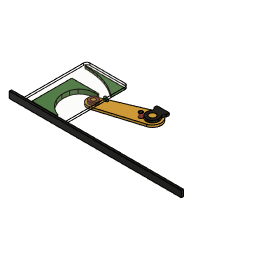
Arpione - Metodo Geometrico [NEW] v2 (Autodesk Fusion 360 design; units mm, degrees)
Autodesk Fusion 360 part; units mm, degrees
sketch "Manovella + Catena" plane through (0, 0, 0) normal (0, 0, 1) x (1, 0, 0)
  circle A0 centre (0, 0) radius 14.5
  line L0 (0, 0) -> (-101.6567, -37)
  circle A1 centre (-101.6567, -37) radius 10
  circle A2 centre (-101.6567, -37) radius 15
  circle A3 centre (0, 0) radius 20.5
  line L1 (-107.497, -23.1837) -> (-7.9817, 18.8823)
  line L2 (-97.2496, -51.338) -> (6.023, -19.5953)
  circle A4 centre (-101.6567, -37) radius 5
  circle A5 centre (0, 0) radius 7.5
  line L3 (-38.7092, -123.6808) -> (196.3889, -123.6808)
  line L4 (-38.7092, -128.6808) -> (196.3889, -128.6808)
  line L5 (196.3889, -128.6808) -> (196.3889, -123.6808)
  line L6 (-99.9998, -123.6808) -> (-207.841, -123.6808)
  line L7 (-207.841, -128.6808) -> (-207.841, -123.6808)
  line L8 (0, 0) -> (6.023, -19.5953) construction
  line L9 (-7.9817, 18.8823) -> (0, 0) construction
  line L10 (0, 0) -> (0, 20.5) construction
  line L11 (-99.9998, -123.6808) -> (-99.9998, -128.6808) construction
  line L12 (-207.841, -128.6808) -> (-99.9998, -128.6808)
  line L13 (-99.9998, -123.6808) -> (-38.7092, -123.6808)
  line L14 (-38.7092, -123.6808) -> (-38.7092, -128.6808) construction
  line L15 (-99.9998, -128.6808) -> (-38.7092, -128.6808)
  line L16 (0, 0) -> (-0.6635, -0.2415)
  line L17 (0, 0) -> (-15.5734, -11.7354)
  circle A6 centre (-15.5734, -11.7354) radius 2.5
  circle A7 centre (-15.5734, -11.7354) radius 4.5
  line L18 (-52.6515, 0) -> (0, 0) construction
  circle A8 centre (-101.6567, -37) radius 13 construction
  line L19 (0, 0) -> (0, -19.5) construction
  circle A9 centre (0, -19.5) radius 4.5 construction
  line L20 (0, -24) -> (-101.6567, -24) construction
  line L21 (-101.6567, -37) -> (-115.7521, -42.1303) construction
  circle A10 centre (0, 0) radius 123.1808 construction
  line L22 (0.0515, -123.1808) -> (0.0515, -123.6808)
  dimension "d1" = 29
  dimension "d8" = 20
  dimension "d43" = 0
  dimension "d44" = 0
  dimension "d45" = 0
  dimension "d46" = 0
  dimension "d197" = 5
  dimension "d198" = 6
  dimension "d199" = -5
  dimension "d200" = -7
  dimension "d312" = 5
  dimension "d449" = 23.372
  dimension "d648" = 19.5
  dimension "d650" = 17
  dimension "d651" = 5
  dimension "d653" = 9
  dimension "d654" = 20
  dimension "d655" = 3
  dimension "d656" = 85.4786
  dimension "d658" = 0.5
  constraint coincident A0.centre L0.start
  constraint coincident L0.end A1.centre
  constraint coincident A2 L1.start
  constraint coincident A3 L1.end
  constraint tangent A3 L1
  constraint tangent A2 L1
  constraint coincident A2 L2.start
  constraint coincident A3 L2.end
  constraint tangent A3 L2
  constraint tangent A2 L2
  constraint perpendicular L3 L5
  constraint coincident L3 L13.end
  constraint horizontal L3
  constraint horizontal L4
  constraint perpendicular L6 L7
  constraint coincident A3 L10.end
  constraint vertical L10
  constraint perpendicular L4 L11
  constraint horizontal L12
  constraint perpendicular L4 L14
  constraint horizontal L15
  constraint coincident L0 L16.end
  constraint coincident L17.end A6.centre
  constraint concentric A6 A7
  constraint horizontal L18
  constraint coincident L1 L18.start
  constraint vertical L19
  constraint equal L17 L19
  constraint coincident L19.end A9.centre
  constraint equal A7 A9
  constraint horizontal L20
  constraint tangent A9 L20
  constraint coincident A9 L20.start
  constraint tangent A8 L20
  constraint coincident A8 L20.end
  constraint coincident A2 L21.end
  constraint collinear L0 L21
  constraint coincident L21.end A10
  constraint coincident A10 L22.start
  constraint coincident L3 L22.end
  constraint perpendicular L3 L22
  measures "d1" diameter of A0
  measures "d8" diameter of A1
  measures "d312" distance of L3.end L4.end
  measures "d540" distance of A0.centre
  measures "d648" distance of A0.centre L17.end
  measures "d650" angle of L0 L17
  measures "d651" diameter of A6
  measures "d653" diameter of A7
  measures "d654" angle of L0 L18
  measures "d658" distance of L22.start L22.end
sketch "Curva Principale" plane through (0, 0, 0) normal (0, 0, 1) x (1, 0, 0)
  circle A0 centre (0, 0) radius 14.5
  circle A1 centre (-101.6567, -37) radius 10
  line L0 (0, 0) -> (-101.6567, -37)
  line L1 (0, 0) -> (-300, 0) construction
  line L2 (-10, 0) -> (-111.5208, -37.3713) construction
  line L3 (-20, 0) -> (-120.62, -39.7327) construction
  line L4 (-30, 0) -> (-128.2041, -45.3766) construction
  line L5 (-40, 0) -> (-133.2404, -54.8571) construction
  line L6 (-50, 0) -> (-134.4276, -67.6392) construction
  line L7 (-60, 0) -> (-130.2578, -82.2613) construction
  line L8 (-70, 0) -> (-119.9523, -95.9575) construction
  line L9 (-80, 0) -> (-103.6726, -105.5589) construction
  circle A2 centre (-111.5208, -37.3713) radius 10 construction
  circle A3 centre (-120.62, -39.7327) radius 10 construction
  circle A4 centre (-128.2041, -45.3766) radius 10 construction
  circle A5 centre (-133.2404, -54.8571) radius 10 construction
  circle A6 centre (-134.4276, -67.6392) radius 10 construction
  circle A7 centre (-130.2578, -82.2613) radius 10 construction
  circle A8 centre (-119.9523, -95.9575) radius 10 construction
  circle A9 centre (-103.6726, -105.5589) radius 10 construction
  line L10 (-165.6808, -117.9148) -> (-165.6808, 0)
  line L11 (-101.6567, -37) -> (-92.2597, -33.5798) construction
  line L12 (-101.6567, -37) -> (-105.0769, -27.6031) construction
  line L13 (-111.5208, -37.3713) -> (-114.9753, -27.9869) construction
  line L14 (-111.5208, -37.3713) -> (-120.9051, -40.8258) construction
  line L15 (-120.62, -39.7327) -> (-129.9211, -43.4055) construction
  line L16 (-120.62, -39.7327) -> (-124.2928, -30.4316) construction
  line L17 (-128.2041, -45.3766) -> (-137.2818, -49.5712) construction
  line L18 (-133.2404, -54.8571) -> (-141.8594, -59.9279) construction
  line L19 (-133.2404, -54.8571) -> (-138.3113, -46.2381) construction
  line L20 (-134.4276, -67.6392) -> (-142.2319, -73.8917) construction
  line L21 (-134.4276, -67.6392) -> (-140.68, -59.8349) construction
  line L22 (-130.2578, -82.2613) -> (-136.7523, -89.8654) construction
  line L23 (-130.2578, -82.2613) -> (-137.8618, -75.7668) construction
  line L24 (-119.9523, -95.9575) -> (-109.1547, -75.2156) construction
  line L25 (-109.1547, -75.2156) -> (-124.5698, -104.8276) construction
  line L26 (-119.9523, -95.9575) -> (-128.8224, -91.34) construction
  line L27 (-103.6726, -105.5589) -> (-105.8608, -115.3166) construction
  line L28 (-103.6726, -105.5589) -> (-113.4302, -103.3707) construction
  line L29 (-128.2041, -45.3766) -> (-132.3986, -36.2989) construction
  line L30 (-102.4867, -27.0345) -> (-102.4867, -23.9148)
  line L31 (-102.4867, -23.9148) -> (-165.6808, -23.9148)
  line L32 (-107.506, -117.9148) -> (-165.6808, -117.9148)
  spline S0 degree 5 poles (-102.4867, -27.0345) (-102.9803, -27.0181) (-103.9715, -26.994) (-105.4699, -26.9842) (-107.4912, -27.0236) (-110.0566, -27.1642) (-112.6596, -27.4066) (-115.2977, -27.7716) (-117.9665, -28.2935) (-120.6573, -29.0126) (-123.3546, -29.9669) (-126.0334, -31.1852) (-128.6561, -32.6772) (-131.1759, -34.4349) (-133.5437, -36.4389) (-135.715, -38.6632) (-137.6558, -41.081) (-139.3501, -43.6698) (-140.7956, -46.4106) (-141.9983, -49.2867) (-142.9681, -52.2823) (-143.7134, -55.3813) (-144.2371, -58.5657) (-144.538, -61.8174) (-144.6118, -65.1181) (-144.4531, -68.4506) (-144.0563, -71.7998) (-143.4169, -75.1531) (-142.532, -78.4992) (-141.4009, -81.8266) (-140.0249, -85.1225) (-138.4082, -88.3709) (-136.5584, -91.5515) (-134.4857, -94.6403) (-132.202, -97.6115) (-129.7196, -100.4395) (-127.0505, -103.101) (-124.2053, -105.5765) (-121.1919, -107.8525) (-118.0161, -109.9209) (-114.6816, -111.7773) (-111.889, -113.0913) (-109.7246, -113.9805) (-108.2507, -114.5306) (-107.506, -114.795) knots 0 0 0 0 0 0 0.025 0.05 0.075 0.1 0.125 0.15 0.175 0.2 0.225 0.25 0.275 0.3 0.325 0.35 0.375 0.4 0.425 0.45 0.475 0.5 0.525 0.55 0.575 0.6 0.625 0.65 0.675 0.7 0.725 0.75 0.775 0.8 0.825 0.85 0.875 0.9 0.925 0.95 0.975 1 1 1 1 1 1
  line L33 (-102.4867, -27.0345) -> (-165.6808, -27.0345) construction
  line L34 (-107.506, -114.795) -> (-107.506, -117.9148)
  line L35 (-107.506, -114.795) -> (-165.6808, -114.795) construction
  line L36 (-102.4867, -27.0345) -> (-101.6567, -37) construction
  line L37 (-112.7142, -27.4428) -> (-111.5208, -37.3713) construction
  line L38 (-135.8335, -38.9121) -> (-128.2041, -45.3766)
  line L39 (-142.8322, -52.029) -> (-133.2404, -54.8571)
  line L40 (-144.4026, -68.3455) -> (-134.4276, -67.6392)
  line L41 (-130.2578, -82.2613) -> (-139.4301, -86.2449)
  line L42 (-119.9523, -95.9575) -> (-126.7298, -103.3105)
  line L43 (-107.506, -114.795) -> (-103.6726, -105.5589)
  point P0 (-10, 0)
  point P1 (-20, 0)
  point P2 (-30, 0)
  point P3 (-40, 0)
  point P4 (-50, 0)
  point P5 (-60, 0)
  point P6 (-70, 0)
  point P7 (-80, 0)
  point P8 (-112.7142, -27.4428)
  point P9 (-124.2928, -30.4316)
  point P10 (-135.8335, -38.9121)
  point P11 (-142.8322, -52.029)
  point P12 (-144.4026, -68.3455)
  point P13 (-139.4301, -86.2449)
  point P14 (-126.7298, -103.3105)
  dimension "d616" = 10
  dimension "d617" = 10
  dimension "d618" = 10
  dimension "d619" = 10
  dimension "d620" = 10
  dimension "d621" = 10
  dimension "d622" = 10
  dimension "d623" = 10
  dimension "d625" = 20
  dimension "d626" = 20.209
  dimension "d627" = 21.548
  dimension "d628" = 24.8
  dimension "d629" = 30.47
  dimension "d630" = 38.7
  dimension "d631" = 49.5
  dimension "d632" = 62.5
  dimension "d633" = 77.36
  dimension "d686" = 94
  constraint coincident A0.centre L0.start
  constraint horizontal L1
  constraint coincident L1 P0
  constraint coincident L1 P1
  constraint coincident L1 P2
  constraint coincident L1 P3
  constraint coincident L1 P4
  constraint coincident L1 P5
  constraint coincident L1 P6
  constraint coincident L1 P7
  constraint coincident P0 L2.start
  constraint coincident P1 L3.start
  constraint coincident P2 L4.start
  constraint coincident P3 L5.start
  constraint coincident P4 L6.start
  constraint coincident P5 L7.start
  constraint coincident P6 L8.start
  constraint coincident P7 L9.start
  constraint equal L0 L2
  constraint equal L2 L3
  constraint equal L3 L4
  constraint equal L4 L5
  constraint equal L5 L6
  constraint equal L6 L7
  constraint equal L7 L8
  constraint equal L8 L9
  constraint coincident L2.end A2.centre
  constraint coincident L3.end A3.centre
  constraint coincident L4.end A4.centre
  constraint coincident L5.end A5.centre
  constraint coincident L6.end A6.centre
  constraint coincident L7.end A7.centre
  constraint coincident L8.end A8.centre
  constraint coincident L9.end A9.centre
  constraint equal A1 A2
  constraint equal A2 A3
  constraint equal A3 A4
  constraint equal A4 A5
  constraint equal A5 A6
  constraint equal A6 A7
  constraint equal A7 A8
  constraint equal A8 A9
  constraint coincident L1 L10.end
  constraint vertical L10
  constraint coincident A1.centre L0.end
  constraint coincident A1 L11.end
  constraint coincident A2 L13.end
  constraint coincident A2 L14.end
  constraint coincident A3 L15.end
  constraint coincident A3 P9
  constraint coincident A4 L17.end
  constraint coincident A5 L18.end
  constraint coincident A5 L19.end
  constraint coincident A6 L20.end
  constraint coincident A6 L21.end
  constraint coincident A7 L22.end
  constraint coincident A7 L23.end
  constraint coincident A8 L25.end
  constraint coincident A8 L26.end
  constraint coincident A9 L27.end
  constraint coincident A9 L28.end
  constraint collinear L0 L11
  constraint collinear L2 L14
  constraint collinear L3 L15
  constraint collinear L4 L17
  constraint collinear L5 L18
  constraint collinear L6 L20
  constraint collinear L7 L22
  constraint collinear L8 L25
  constraint collinear L9 L27
  constraint perpendicular L27 L28
  constraint perpendicular L25 L26
  constraint perpendicular L22 L23
  constraint perpendicular L20 L21
  constraint perpendicular L18 L19
  constraint perpendicular L15 L16
  constraint coincident A4 L29.end
  constraint perpendicular L17 L29
  constraint perpendicular L13 L14
  constraint perpendicular L11 L12
  constraint coincident L10 L31.end
  constraint perpendicular L10 L31
  constraint coincident L10.start L32.end
  constraint coincident A1 L12.end
  constraint coincident A2 P8
  constraint coincident A4 P10
  constraint coincident A5 P11
  constraint coincident A6 P12
  constraint coincident A7 P13
  constraint coincident A8 P14
  constraint coincident A9 S0.end
  constraint coincident A1 L30.start
  constraint coincident L10 L33.end
  constraint perpendicular L10 L33
  constraint perpendicular L32 L34
  constraint coincident L10 L35.end
  constraint perpendicular L10 L35
  constraint equal L30 L34
  constraint vertical L30
  constraint vertical L34
  constraint coincident P8 L37.start
  constraint coincident P10 L38.start
  constraint coincident P11 L39.start
  constraint coincident P12 L40.start
  constraint coincident P13 L41.end
  constraint coincident P14 L42.end
  measures "d616" distance of A0.centre P0
  measures "d617" distance of P0 P1
  measures "d618" distance of P1 P2
  measures "d619" distance of P2 P3
  measures "d620" distance of P3 P4
  measures "d621" distance of P4 P5
  measures "d622" distance of P5 P6
  measures "d623" distance of P6 P7
  measures "d625" angle of L0 L1
  measures "d626" angle of L1 L2
  measures "d627" angle of L1 L3
  measures "d628" angle of L1 L4
  measures "d629" angle of L1 L5
  measures "d630" angle of L1 L6
  measures "d631" angle of L1 L7
  measures "d632" angle of L1 L8
  measures "d633" angle of L1 L9
  measures "d686" distance of L10.start L31.end
sketch "Curva secondaria" plane through (0, 0, 0) normal (0, 0, 1) x (1, 0, 0)
  line L0 (-100.0056, -0.0109) -> (0, 0.0109)
  circle A0 centre (-88.1799, -15.52) radius 4.5 construction
  line L1 (-80, 0) -> (-78.5176, -19.4436) construction
  circle A1 centre (-78.5176, -19.4436) radius 4.5 construction
  line L2 (-88.1799, -15.52) -> (-100, -0.0109) construction
  line L3 (-80, 0) -> (-103.6726, -105.5589)
  circle A2 centre (-103.6726, -105.5589) radius 10
  line L4 (-90, -0.0087) -> (-83.167, -18.2723) construction
  circle A3 centre (-83.167, -18.2723) radius 4.5 construction
  line L5 (-91.4991, -20.02) -> (-88.1799, -20.02) construction
  line L6 (-91.4815, -23.9436) -> (-78.5176, -23.9436) construction
  circle A4 centre (-15.5734, -11.7354) radius 4.5
  line L7 (0, 0) -> (-15.5734, -11.7354)
  line L8 (-91.5063, -22.7723) -> (-83.167, -22.7723) construction
  line L9 (-83.167, -18.2723) -> (-81.5901, -22.487) construction
  line L10 (-83.167, -18.2723) -> (-87.3817, -19.8492) construction
  line L11 (-88.1799, -15.52) -> (-85.4521, -19.0991) construction
  line L12 (-88.1799, -15.52) -> (-91.7589, -18.2478) construction
  arc A5 (-89.8544, -20.02) -> (-79.0195, -23.9436) centre (-84.6752, -22.6399) ccw
  line L13 (-89.8544, -20.02) -> (-84.2048, -22.7723)
  line L14 (-84.2048, -22.7723) -> (-79.0195, -23.9436)
  line L15 (-78.5176, -19.4436) -> (-78.1754, -23.9305) construction
  line L16 (-78.5176, -19.4436) -> (-83.0045, -19.7857) construction
  point P0 (-100, -0.0109)
  point P1 (-90, -0.0087)
  dimension "d536" = 127.3
  dimension "d638" = 73.708
  dimension "d639" = 10
  dimension "d641" = 10
  dimension "d642" = 110.5
  dimension "d649" = 17
  dimension "d657" = 36.988
  constraint coincident L1.end A1.centre
  constraint coincident L1.start L3.start
  constraint coincident A0.centre L2.start
  constraint coincident P0 L2.end
  constraint coincident L0 P0
  constraint coincident L0 P1
  constraint coincident P1 L4.start
  constraint equal L1 L4
  constraint coincident L4.end A3.centre
  constraint equal A1 A3
  constraint equal A0 A3
  constraint equal L2 L4
  constraint horizontal L5
  constraint horizontal L6
  constraint tangent A1 L6
  constraint tangent A0 L5
  constraint horizontal L8
  constraint tangent A3 L8
  constraint coincident A3 L8.end
  constraint coincident A0 L5.end
  constraint coincident A1 L6.end
  constraint coincident A3 L9.end
  constraint parallel L4 L9
  constraint coincident A3 L10.end
  constraint perpendicular L9 L10
  constraint coincident A0 L11.end
  constraint collinear L2 L11
  constraint coincident A0 L12.end
  constraint perpendicular L11 L12
  constraint coincident L6 A5.end
  constraint equal A1 A4
  constraint equal L1 L7
  constraint coincident L5 A5.start
  constraint coincident L8 L13.end
  constraint tangent A3 L13
  constraint tangent A1 L14
  constraint coincident A1 L15.end
  constraint coincident A1 L16.end
  constraint perpendicular L1 L16
  measures "d536" angle of L0 L2
  measures "d639" horizontal distance of L1.start P1
  measures "d641" horizontal distance of P0 P1
  measures "d642" angle of L0 L4
  measures "d649" angle of L1 L3
  measures "d657" angle of L0 L7
extrude "Extrude1" add sketch "Curva Principale" along normal blind 10 contours L10 L30 L31 L32 S0 L34 makes body 1 in component "Arpione_Curva1"
fillet "Fillet12" radius 0.4 2 edges at (-102.4867, -27.0345, 5) (-107.506, -114.795, 5) on bodies 1 in component "Arpione_Curva1"
extrude "Extrude1'" add sketch "Manovella + Catena" against normal blind 5 separate body contours A0 L0 A5 L17 | A0 L0 A3 L17 A7 | A0 L0 A5 L17 | A0 L0 A3 L17 A7 | L0 A5 L16 L17 | L0 A5 L16 L17 | L0 A2 A3 L2 A7 | L0 A2 A3 L1 | A3 L17 A6 A7 | A3 L17 A6 A7 | A2 | A3 A6 A7 | A3 A6 | A3 A6 | A1 | A4 makes body 2 in component "Manopola"
extrude "Extrude2" add sketch "Manovella + Catena" along normal blind 5 contours A4 bodies 2 in component "Manopola"
extrude "Extrude3" add sketch "Manovella + Catena" against normal blind 10 contours L0 A5 L16 L17 | L0 A5 L16 L17 bodies 2 in component "Manopola"
extrude "Extrude4" add sketch "Manovella + Catena" along normal blind 10 contours A3 A6 | A3 A6 bodies 2 in component "Manopola"
extrude "Extrude5" add sketch "Manovella + Catena" along normal blind 5 contours L0 A5 L16 L17 | L0 A5 L16 L17 bodies 2 in component "Manopola"
sketch "Fulcro" plane through (0, 0, 0) normal (0, 0, 1) x (1, 0, 0)
  circle A0 centre (0, 0) radius 14.5
  circle A1 centre (0, 0) radius 7.5
  line L0 (0, 0) -> (-14.5, 0)
  line L1 (0, 0) -> (14.5, 0)
  line L2 (14.5, 0) -> (14.5, 25)
  line L3 (14.5, 25) -> (-14.5, 25)
  line L4 (-14.5, 25) -> (-14.5, 0)
  line L5 (-15.5734, -11.7354) -> (0, 0)
  line L6 (0, 0) -> (15.5734, 11.7354) construction
  circle A2 centre (15.5734, 11.7354) radius 4.5 construction
  arc A3 (14.5, 17.9188) -> (14.5, 6.5018) centre (17.4303, 12.2103) ccw
  line L7 (0, 0) -> (0, 14.5) construction
  circle A4 centre (-15.5734, -11.7354) radius 4.5
  arc A5 (14.5, 0) -> (12.1494, 8.5653) centre (-2.2808, 0) ccw
  arc A6 (-14.5, 6.5018) -> (-14.5, 17.9188) centre (-17.4303, 12.2103) ccw
  arc A7 (-12.1494, 8.5653) -> (-14.5, 0) centre (2.2808, 0) ccw
  dimension "d540" = 25
  constraint coincident A0.centre A1.centre
  constraint coincident A0 L0.end
  constraint horizontal L0
  constraint coincident A0 L1.end
  constraint horizontal L1
  constraint perpendicular L1 L2
  constraint perpendicular L2 L3
  constraint tangent A0 L4
  constraint coincident L5.start A4.centre
  constraint parallel L5 L6
  constraint equal L5 L6
  constraint coincident L6.end A2.centre
  constraint equal A2 A4
  constraint tangent A2 A3
  constraint coincident L2 A3.end
  constraint coincident L2 A3.start
  constraint coincident A0 L7.end
  constraint vertical L7
  constraint tangent L2 A5
  constraint coincident A3 A5.end
  constraint symmetric L1.end L7 L0.end
  constraint symmetric A3.start L7 A6.end
  constraint symmetric A3.end L7 A6.start
  constraint symmetric A3 L7 A6
  constraint symmetric L7 A5.end A7.start
  constraint symmetric L7 A5 A7
  measures "d540" distance of L1.end L2.end
extrude "Extrude1''" add sketch "Fulcro" along normal blind 5 separate body contours A0 A1 L0 L1 | A0 A1 L1 L5 | A0 L2 L3 L4 A3 A5 A6 A7 | A0 A1 L0 L5 makes body 3 in component "Fulcro"
extrude "Extrude1'''" add sketch "Manovella + Catena" along normal blind 5 separate body contours A1 makes body 4 in component "Cuscinetto_Basso"
extrude "Extrude1''''" add sketch "Manovella + Catena" along normal blind 10 separate body contours A3 L17 A6 A7 | A3 L17 A6 A7 | A3 A6 A7 makes body 5 in component "Cuscinetto_Alto"
extrude "Extrude1'''''" add sketch "Manovella + Catena" along normal blind 15 separate body contours L3 L4 L5 L6 L7 L12 L13 L15 makes body 6 in component "Catena"
extrude "Extrude1''''''" add sketch "Curva secondaria" along normal blind 4 from surface at 6 separate body contours L3 A5 L13 L14 | L3 A5 L13 makes body 7 in component "Arpione_Curva2"
sketch "Curva Frenante" plane through (0, 0, 0) normal (0, 0, 1) x (1, 0, 0)
  circle A0 centre (0, 0) radius 14.5
  line L0 (-88.1799, -15.52) -> (-100, -0.0109) construction
  circle A1 centre (-88.1799, -15.52) radius 4.5
  line L1 (0, 0) -> (-300, 0) construction
  line L2 (-110, 0) -> (-94.2042, -11.4343) construction
  line L3 (-120, 0) -> (-101.6528, -6.6054) construction
  line L4 (-130, 0) -> (-110.5713, -1.6656) construction
  line L5 (-140, 0) -> (-120.6898, 2.7139) construction
  line L6 (-150, 0) -> (-131.5294, 6.252) construction
  line L7 (-160, 0) -> (-142.6099, 8.8225) construction
  line L8 (-170, 0) -> (-153.5539, 10.4773) construction
  line L9 (-180, 0) -> (-164.1644, 11.3791) construction
  line L10 (-190, 0) -> (-174.4061, 11.7082) construction
  circle A2 centre (-94.2042, -11.4343) radius 4.5 construction
  circle A3 centre (-101.6528, -6.6054) radius 4.5 construction
  circle A4 centre (-110.5713, -1.6656) radius 4.5 construction
  circle A5 centre (-120.6898, 2.7139) radius 4.5 construction
  circle A6 centre (-131.5294, 6.252) radius 4.5 construction
  circle A7 centre (-142.6099, 8.8225) radius 4.5 construction
  circle A8 centre (-153.5539, 10.4773) radius 4.5 construction
  circle A9 centre (-164.1644, 11.3791) radius 4.5 construction
  circle A10 centre (-174.4061, 11.7082) radius 4.5 construction
  circle A11 centre (-15.5734, -11.7354) radius 4.5
  line L11 (0, 0) -> (-15.5734, -11.7354)
  line L12 (-88.1799, -15.52) -> (-84.6008, -12.7923)
  line L13 (-94.2042, -11.4343) -> (-91.5655, -7.7891) construction
  line L14 (-101.6528, -6.6054) -> (-100.1285, -2.3714)
  line L15 (-110.5713, -1.6656) -> (-110.1869, 2.8179)
  line L16 (-120.6898, 2.7139) -> (-121.3161, 7.1701)
  line L17 (-131.5294, 6.252) -> (-132.9722, 10.5144)
  line L18 (-142.6099, 8.8225) -> (-144.6459, 12.8356)
  line L19 (-153.5539, 10.4773) -> (-155.9717, 14.2726)
  line L20 (-164.1644, 11.3791) -> (-166.7903, 15.0334)
  line L21 (-174.4061, 11.7082) -> (-177.108, 15.3068)
  line L22 (-174.4061, 11.7082) -> (-170.8076, 14.4101)
  line L23 (-164.1644, 11.3791) -> (-160.51, 14.005)
  line L24 (-153.5539, 10.4773) -> (-149.7586, 12.8952)
  line L25 (-142.6099, 8.8225) -> (-138.5969, 10.8584)
  line L26 (-131.5294, 6.252) -> (-127.267, 7.6947)
  line L27 (-120.6898, 2.7139) -> (-116.2336, 3.3402)
  line L28 (-110.5713, -1.6656) -> (-106.0877, -2.05)
  line L29 (-101.6528, -6.6054) -> (-97.4189, -8.1297)
  line L30 (-174.3889, 18.1861) -> (-84.3889, 18.1861)
  line L31 (-84.3889, 18.1861) -> (-84.3889, -11.8139)
  line L32 (-94.2042, -11.4343) -> (-90.559, -14.0729)
  line L33 (-88.1799, -15.52) -> (-85.4521, -19.0991)
  line L34 (-174.3889, 18.1861) -> (-174.3889, 16.2082)
  line L35 (-85.6275, -11.8139) -> (-84.3889, -11.8139)
  spline S0 degree 5 poles (-85.6275, -11.8139) (-85.8881, -11.6362) (-86.4153, -11.2768) (-87.2243, -10.7261) (-88.3396, -9.9682) (-89.7941, -8.9825) (-91.3079, -7.9606) (-92.878, -6.9074) (-94.4996, -5.8312) (-96.1662, -4.7426) (-97.8716, -3.6529) (-99.6106, -2.5729) (-101.38, -1.5111) (-103.18, -0.4727) (-105.0128, 0.5398) (-106.8812, 1.5253) (-108.7879, 2.4837) (-110.734, 3.4149) (-112.7184, 4.3181) (-114.7379, 5.192) (-116.7885, 6.035) (-118.8654, 6.8454) (-120.964, 7.6217) (-123.0804, 8.3627) (-125.2113, 9.0674) (-127.3537, 9.7352) (-129.505, 10.3659) (-131.6627, 10.9592) (-133.8242, 11.5155) (-135.9867, 12.035) (-138.1479, 12.5184) (-140.306, 12.9665) (-142.4599, 13.3802) (-144.6097, 13.7605) (-146.7567, 14.1086) (-148.9025, 14.4256) (-151.0491, 14.7129) (-153.1975, 14.9716) (-155.3478, 15.2031) (-157.4984, 15.4084) (-159.6466, 15.5887) (-161.7893, 15.745) (-163.9232, 15.878) (-166.0455, 15.9886) (-168.1544, 16.0771) (-170.2488, 16.144) (-171.9124, 16.1803) (-173.1533, 16.198) (-173.9775, 16.2055) (-174.3889, 16.2082) knots 0 0 0 0 0 0 0.022222 0.044444 0.066667 0.088889 0.111111 0.133333 0.155556 0.177778 0.2 0.222222 0.244444 0.266667 0.288889 0.311111 0.333333 0.355556 0.377778 0.4 0.422222 0.444444 0.466667 0.488889 0.511111 0.533333 0.555556 0.577778 0.6 0.622222 0.644444 0.666667 0.688889 0.711111 0.733333 0.755556 0.777778 0.8 0.822222 0.844444 0.866667 0.888889 0.911111 0.933333 0.955556 0.977778 1 1 1 1 1 1
  line L36 (-85.6275, -11.8139) -> (-88.1799, -15.52)
  line L37 (-99.4248, -2.6957) -> (-101.6528, -6.6054)
  line L38 (-108.5716, 2.3657) -> (-110.5713, -1.6656)
  line L39 (-119.0916, 6.9205) -> (-120.6898, 2.7139)
  line L40 (-130.4406, 10.6182) -> (-131.5294, 6.252)
  line L41 (-141.8259, 13.2536) -> (-142.6099, 8.8225)
  line L42 (-152.9365, 14.9348) -> (-153.5539, 10.4773)
  line L43 (-163.9305, 15.873) -> (-164.1644, 11.3791)
  line L44 (-174.3889, 16.2082) -> (-174.4061, 11.7082)
  point P0 (-110, 0)
  point P1 (-120, 0)
  point P2 (-130, 0)
  point P3 (-140, 0)
  point P4 (-150, 0)
  point P5 (-160, 0)
  point P6 (-170, 0)
  point P7 (-180, 0)
  point P8 (-190, 0)
  point P9 (-91.5655, -7.7891)
  point P10 (-99.4248, -2.6957)
  point P11 (-108.5716, 2.3657)
  point P12 (-119.0916, 6.9205)
  point P13 (-130.4406, 10.6182)
  point P14 (-141.8259, 13.2536)
  point P15 (-152.9365, 14.9348)
  point P16 (-163.9305, 15.873)
  dimension "d558" = 10
  dimension "d563" = 10
  dimension "d567" = 115.112
  dimension "d568" = 144.1
  dimension "d569" = 160.2
  dimension "d570" = 175.1
  dimension "d571" = 188
  dimension "d572" = 198.7
  dimension "d573" = 206.9
  dimension "d574" = 212.5
  dimension "d575" = 215.7
  dimension "d576" = 216.9
  dimension "d661" = 10
  dimension "d662" = 10
  dimension "d663" = 10
  dimension "d664" = 10
  dimension "d665" = 10
  dimension "d666" = 10
  dimension "d667" = 10
  dimension "d688" = 90
  dimension "d689" = 30
  constraint coincident A0.centre L1.start
  constraint coincident L1 P0
  constraint coincident L1 P1
  constraint coincident L1 P2
  constraint coincident L1 P3
  constraint coincident L1 P4
  constraint coincident L1 P5
  constraint coincident L1 P6
  constraint coincident L1 P7
  constraint coincident L1 P8
  constraint coincident P0 L2.start
  constraint coincident P1 L3.start
  constraint coincident P2 L4.start
  constraint coincident P3 L5.start
  constraint coincident P4 L6.start
  constraint coincident P5 L7.start
  constraint coincident P6 L8.start
  constraint coincident P7 L9.start
  constraint coincident P8 L10.start
  constraint equal L0 L2
  constraint equal L2 L3
  constraint equal L3 L4
  constraint equal L4 L5
  constraint equal L5 L6
  constraint equal L6 L7
  constraint equal L7 L8
  constraint equal L8 L9
  constraint equal L9 L10
  constraint coincident L2.end A2.centre
  constraint coincident L3.end A3.centre
  constraint coincident L4.end A4.centre
  constraint coincident L5.end A5.centre
  constraint coincident L6.end A6.centre
  constraint coincident L7.end A7.centre
  constraint coincident L8.end A8.centre
  constraint coincident L9.end A9.centre
  constraint coincident L10.end A10.centre
  constraint equal A1 A2
  constraint equal A2 A3
  constraint equal A3 A4
  constraint equal A4 A5
  constraint equal A5 A6
  constraint equal A6 A7
  constraint equal A7 A8
  constraint equal A8 A9
  constraint equal A9 A10
  constraint coincident L0.start A1.centre
  constraint coincident A1 L35.start
  constraint coincident A2 P9
  constraint coincident A3 L14.end
  constraint perpendicular L3 L14
  constraint coincident A4 L15.end
  constraint perpendicular L4 L15
  constraint coincident A5 L16.end
  constraint perpendicular L5 L16
  constraint coincident A6 L17.end
  constraint perpendicular L6 L17
  constraint coincident A7 L18.end
  constraint perpendicular L7 L18
  constraint coincident A8 L19.end
  constraint perpendicular L8 L19
  constraint coincident A9 L20.end
  constraint perpendicular L9 L20
  constraint coincident A10 L21.end
  constraint perpendicular L10 L21
  constraint coincident A10 L22.end
  constraint perpendicular L21 L22
  constraint coincident A9 L23.end
  constraint perpendicular L20 L23
  constraint coincident A8 L24.end
  constraint perpendicular L19 L24
  constraint coincident A7 L25.end
  constraint perpendicular L18 L25
  constraint coincident A6 L26.end
  constraint perpendicular L17 L26
  constraint coincident A5 L27.end
  constraint perpendicular L16 L27
  constraint coincident A4 L28.end
  constraint perpendicular L15 L28
  constraint coincident A3 L29.end
  constraint perpendicular L14 L29
  constraint perpendicular L2 L13
  constraint perpendicular L0 L12
  constraint coincident A2 L32.end
  constraint perpendicular L13 L32
  constraint coincident A1 L33.end
  constraint perpendicular L12 L33
  constraint coincident A10 L34.end
  constraint perpendicular L30 L34
  constraint horizontal L30
  constraint vertical L31
  constraint perpendicular L31 L35
  constraint coincident A3 P10
  constraint coincident A4 P11
  constraint coincident A5 P12
  constraint coincident A6 P13
  constraint coincident A7 P14
  constraint coincident A8 P15
  constraint coincident A9 P16
  constraint coincident P10 L37.start
  constraint coincident P11 L38.start
  constraint coincident P12 L39.start
  constraint coincident P13 L40.start
  constraint coincident P14 L41.start
  constraint coincident P15 L42.start
  constraint coincident P16 L43.start
  measures "d558" horizontal distance of L0.end P0
  measures "d563" distance of P4 P5
  measures "d568" angle of L1 L2
  measures "d569" angle of L1 L3
  measures "d570" angle of L1 L4
  measures "d661" distance of P0 P1
  measures "d662" distance of P1 P2
  measures "d663" distance of P2 P3
  measures "d664" distance of P3 P4
  measures "d665" distance of P5 P6
  measures "d666" distance of P7 P6
  measures "d667" distance of P8 P7
  measures "d688" distance of L30.start L30.end
  measures "d689" distance of L31.end L30.end
extrude "Extrude1'''''''" add sketch "Curva Frenante" along normal blind 5 from surface at 5 separate body contours L30 L31 L34 L35 S0 makes body 8 in component "Arpione_Curva3"
move_body "Move1" bodies 8 to x (1, 0, 0) y (0, 1, 0) z (0, 0, 1) at (-0.65, 0, 0) in component "Arpione_Curva3"
fillet "Fillet2" radius 0.3 2 edges at (-86.2775, -11.8139, 7.5) (-175.0389, 16.2082, 7.5) on bodies 8 in component "Arpione_Curva3"
sketch "Struttura" plane through (0, 0, 0) normal (0, 0, 1) x (1, 0, 0)
  line L0 (-102.4867, -26.6222) -> (-102.4867, -23.9148) construction
  line L1 (-102.4867, -23.9148) -> (-165.6808, -23.9148) construction
  line L2 (-165.6808, -23.9148) -> (-165.6808, -117.9148) construction
  line L3 (-165.6808, -117.9148) -> (-107.506, -117.9148) construction
  line L4 (-85.0389, -11.8139) -> (-85.0389, 18.1861) construction
  line L5 (-85.0389, 18.1861) -> (-175.0389, 18.1861) construction
  line L6 (-207.841, -128.6808) -> (196.3889, -128.6808)
  line L7 (196.3889, -128.6808) -> (196.3889, -123.6808)
  line L8 (196.3889, -123.6808) -> (-207.841, -123.6808)
  line L9 (-207.841, -123.6808) -> (-207.841, -128.6808)
  line L10 (-165.6808, -23.9148) -> (-165.6808, 18.1881) construction
  line L11 (-165.6808, 18.1881) -> (-175.0389, 18.1861)
  line L12 (-85.0389, -11.8139) -> (-85.0389, -123.6808) construction
  line L13 (-165.6808, -117.9148) -> (-165.6808, -123.6808) construction
  line L14 (-80.0389, -123.6808) -> (-80.0389, 15.6861)
  line L15 (-87.5389, 23.1861) -> (-170.1808, 23.1861)
  line L16 (-130.0389, 18.1861) -> (-130.0389, -123.6808) construction
  line L17 (-177.6808, 15.6861) -> (-177.6808, -123.6808)
  arc A0 (-170.1808, 23.1861) -> (-177.6808, 15.6861) centre (-170.1808, 15.6861) ccw
  arc A1 (-80.0389, 15.6861) -> (-87.5389, 23.1861) centre (-87.5389, 15.6861) ccw
  arc A2 (-89.8544, -20.02) -> (-79.0195, -23.9436) centre (-84.6752, -22.6399) ccw
  spline S0 degree 5 poles (-135.8335, -38.9121) (-135.7985, -38.8718) (-135.3555, -38.3654) (-134.4788, -37.4144) (-133.1109, -36.0726) (-131.1759, -34.4349) (-128.6561, -32.6772) (-126.0334, -31.1852) (-123.3546, -29.9669) (-120.6573, -29.0126) (-117.9665, -28.2935) (-115.2977, -27.7716) (-112.6596, -27.4066) (-110.0566, -27.1642) (-107.5765, -27.0283) (-105.638, -26.9876) (-104.2208, -26.9928) (-103.3102, -27.0108) (-102.8976, -27.0221) knots -0.327153 -0.327153 -0.327153 -0.327153 -0.327153 -0.327153 -0.325 -0.3 -0.275 -0.25 -0.225 -0.2 -0.175 -0.15 -0.125 -0.1 -0.075 -0.05 -0.025 -0.004157 -0.004157 -0.004157 -0.004157 -0.004157 -0.004157
  line L18 (-107.506, -117.9148) -> (-107.506, -115.0768)
  spline S1 degree 5 poles (-107.7705, -114.7004) (-108.4602, -114.4521) (-109.8785, -113.9171) (-111.9883, -113.0445) (-114.7291, -111.7509) (-118.0161, -109.9209) (-121.1283, -107.8939) (-123.4819, -106.1227) (-125.1614, -104.7216) (-126.2305, -103.7692) (-126.7298, -103.3105) knots -0.998222 -0.998222 -0.998222 -0.998222 -0.998222 -0.998222 -0.975 -0.95 -0.925 -0.9 -0.875 -0.852502 -0.852502 -0.852502 -0.852502 -0.852502 -0.852502
  spline S2 degree 5 poles (-126.7298, -103.3105) (-126.7853, -103.2595) (-127.3946, -102.6978) (-128.5376, -101.6039) (-130.1664, -99.9305) (-132.202, -97.6115) (-134.4857, -94.6403) (-136.4143, -91.7664) (-137.7796, -89.4489) (-138.6895, -87.7411) (-139.2241, -86.6692) (-139.4301, -86.2449) knots -0.852502 -0.852502 -0.852502 -0.852502 -0.852502 -0.852502 -0.85 -0.825 -0.8 -0.775 -0.75 -0.725 -0.708694 -0.708694 -0.708694 -0.708694 -0.708694 -0.708694
  spline S3 degree 5 poles (-139.4301, -86.2449) (-139.5399, -86.0187) (-139.9599, -85.1406) (-140.6539, -83.6027) (-141.5484, -81.3926) (-142.532, -78.4992) (-143.4169, -75.1531) (-143.9326, -72.4485) (-144.2089, -70.4165) (-144.3446, -69.0571) (-144.4008, -68.3673) (-144.4026, -68.3455) knots -0.708694 -0.708694 -0.708694 -0.708694 -0.708694 -0.708694 -0.7 -0.675 -0.65 -0.625 -0.6 -0.575 -0.574181 -0.574181 -0.574181 -0.574181 -0.574181 -0.574181
  spline S4 degree 5 poles (-144.4026, -68.3455) (-144.4549, -67.6995) (-144.5387, -66.3874) (-144.5961, -64.4147) (-144.536, -61.7961) (-144.2371, -58.5657) (-143.8085, -55.9597) (-143.3788, -54.0314) (-143.0391, -52.7483) (-142.8483, -52.0847) (-142.8322, -52.029) knots -0.574181 -0.574181 -0.574181 -0.574181 -0.574181 -0.574181 -0.55 -0.525 -0.5 -0.475 -0.45 -0.447705 -0.447705 -0.447705 -0.447705 -0.447705 -0.447705
  spline S5 degree 5 poles (-142.8322, -52.029) (-142.6726, -51.4775) (-142.3176, -50.3277) (-141.7135, -48.6059) (-140.769, -46.3603) (-139.375, -43.717) (-138.0529, -41.688) (-136.964, -40.2498) (-136.2054, -39.339) (-135.8335, -38.9121) knots -0.447705 -0.447705 -0.447705 -0.447705 -0.447705 -0.447705 -0.425 -0.4 -0.375 -0.35 -0.327153 -0.327153 -0.327153 -0.327153 -0.327153 -0.327153
  spline S6 degree 3 poles (-107.7705, -114.7004) (-107.7215, -114.7181) (-107.6764, -114.7451) (-107.5991, -114.815) (-107.5677, -114.8571) (-107.5323, -114.931) (-107.5225, -114.9592) (-107.5093, -115.0173) (-107.506, -115.047) (-107.506, -115.0768) knots 0 0 0 0 0.015626 0.015626 0.031252 0.031252 0.040187 0.040187 0.049122 0.049122 0.049122 0.049122
  spline S7 degree 3 poles (-102.4867, -26.6222) (-102.4867, -26.6743) (-102.4969, -26.7259) (-102.5364, -26.8223) (-102.5654, -26.8661) (-102.6386, -26.9403) (-102.6821, -26.9698) (-102.7564, -27.0015) (-102.7839, -27.0099) (-102.8403, -27.0206) (-102.8689, -27.0229) (-102.8976, -27.0221) knots 0 0 0 0 0.015626 0.015626 0.031252 0.031252 0.046877 0.046877 0.055482 0.055482 0.064086 0.064086 0.064086 0.064086
  line L19 (-79.0195, -23.9436) -> (-84.2048, -22.7723)
  line L20 (-84.2048, -22.7723) -> (-89.8544, -20.02)
  line L21 (-86.1961, -11.8139) -> (-85.0389, -11.8139)
  line L22 (-175.0389, 18.1861) -> (-175.0389, 16.506)
  spline S8 degree 5 poles (-174.7413, 16.206) (-174.389, 16.2032) (-173.6238, 16.1953) (-172.4421, 16.1777) (-170.8383, 16.142) (-168.8064, 16.0772) (-167.1213, 16.0064) (-165.852, 15.9435) (-165.0041, 15.8972) (-164.5805, 15.873) knots -0.996786 -0.996786 -0.996786 -0.996786 -0.996786 -0.996786 -0.977778 -0.955556 -0.933333 -0.911111 -0.888996 -0.888996 -0.888996 -0.888996 -0.888996 -0.888996
  spline S9 degree 5 poles (-164.5805, 15.873) (-164.5785, 15.8729) (-164.1509, 15.8484) (-163.2965, 15.7973) (-162.0128, 15.7139) (-160.2966, 15.5887) (-158.1484, 15.4084) (-156.3756, 15.2392) (-155.033, 15.0983) (-154.1209, 14.9964) (-153.6388, 14.9408) (-153.5865, 14.9348) knots -0.888996 -0.888996 -0.888996 -0.888996 -0.888996 -0.888996 -0.888889 -0.866667 -0.844444 -0.822222 -0.8 -0.777778 -0.775074 -0.775074 -0.775074 -0.775074 -0.775074 -0.775074
  spline S10 degree 5 poles (-153.5865, 14.9348) (-153.209, 14.8911) (-152.4018, 14.7955) (-151.1653, 14.6414) (-149.5003, 14.4179) (-147.4067, 14.1086) (-145.5628, 13.8096) (-144.1468, 13.5628) (-143.1597, 13.3823) (-142.6025, 13.2776) (-142.4759, 13.2536) knots -0.775074 -0.775074 -0.775074 -0.775074 -0.775074 -0.775074 -0.755556 -0.733333 -0.711111 -0.688889 -0.666667 -0.660132 -0.660132 -0.660132 -0.660132 -0.660132 -0.660132
  spline S11 degree 5 poles (-142.4759, 13.2536) (-142.1719, 13.1962) (-141.4371, 13.0553) (-140.2705, 12.8241) (-138.6708, 12.49) (-136.6367, 12.035) (-134.6616, 11.5605) (-133.1196, 11.1666) (-132.0111, 10.8708) (-131.335, 10.6858) (-131.0906, 10.6182) knots -0.660132 -0.660132 -0.660132 -0.660132 -0.660132 -0.660132 -0.644444 -0.622222 -0.6 -0.577778 -0.555556 -0.542962 -0.542962 -0.542962 -0.542962 -0.542962 -0.542962
  spline S12 degree 5 poles (-131.0906, 10.6182) (-130.9037, 10.5666) (-130.2856, 10.3946) (-129.2372, 10.0962) (-127.7609, 9.6595) (-125.8613, 9.0674) (-123.7754, 8.3776) (-122.1268, 7.8012) (-120.9089, 7.358) (-120.1154, 7.0618) (-119.7416, 6.9205) knots -0.542962 -0.542962 -0.542962 -0.542962 -0.542962 -0.542962 -0.533333 -0.511111 -0.488889 -0.466667 -0.444444 -0.424571 -0.424571 -0.424571 -0.424571 -0.424571 -0.424571
  spline S13 degree 5 poles (-119.7416, 6.9205) (-119.6974, 6.9038) (-119.2354, 6.729) (-118.3581, 6.3921) (-117.0717, 5.8842) (-115.3879, 5.192) (-113.3684, 4.3181) (-111.7343, 3.5743) (-110.5156, 2.9975) (-109.6965, 2.5996) (-109.2667, 2.3879) (-109.2216, 2.3657) knots -0.424571 -0.424571 -0.424571 -0.424571 -0.424571 -0.424571 -0.422222 -0.4 -0.377778 -0.355556 -0.333333 -0.311111 -0.308499 -0.308499 -0.308499 -0.308499 -0.308499 -0.308499
  spline S14 degree 5 poles (-109.2216, 2.3657) (-108.8824, 2.1983) (-108.1621, 1.8392) (-107.0697, 1.2818) (-105.6197, 0.516) (-103.83, -0.4727) (-102.3502, -1.3263) (-101.2453, -1.9836) (-100.5024, -2.434) (-100.1135, -2.672) (-100.0748, -2.6957) knots -0.308499 -0.308499 -0.308499 -0.308499 -0.308499 -0.308499 -0.288889 -0.266667 -0.244444 -0.222222 -0.2 -0.197547 -0.197547 -0.197547 -0.197547 -0.197547 -0.197547
  spline S15 degree 5 poles (-100.0748, -2.6957) (-99.7633, -2.8864) (-99.1044, -3.2931) (-98.1053, -3.919) (-96.7794, -4.7666) (-95.1496, -5.8312) (-93.528, -6.9074) (-91.9579, -7.9606) (-90.4441, -8.9825) (-88.9971, -9.9631) (-87.8887, -10.7163) (-87.0862, -11.2626) (-86.5653, -11.6176) (-86.3112, -11.7909) knots -0.197547 -0.197547 -0.197547 -0.197547 -0.197547 -0.197547 -0.177778 -0.155556 -0.133333 -0.111111 -0.088889 -0.066667 -0.044444 -0.022222 -0.000574 -0.000574 -0.000574 -0.000574 -0.000574 -0.000574
  spline S16 degree 3 poles (-174.7413, 16.206) (-174.7803, 16.2063) (-174.819, 16.2142) (-174.891, 16.2445) (-174.9237, 16.2665) (-174.9789, 16.3218) (-175.0008, 16.3546) (-175.031, 16.4272) (-175.0389, 16.4664) (-175.0389, 16.506) knots 0 0 0 0 0.011719 0.011719 0.023439 0.023439 0.035158 0.035158 0.047032 0.047032 0.047032 0.047032
  arc A3 (-86.3112, -11.7909) -> (-86.1961, -11.8139) centre (-86.1961, -11.5139) ccw
  line L23 (-177.6808, -123.6808) -> (-207.841, -123.6808)
  point P0 (-80.0389, -123.6808)
  dimension "d675" = 5
  dimension "d676" = 5
  dimension "d677" = 12
  dimension "d678" = 7.5
  constraint coincident L1.end L2.start
  constraint perpendicular L5 L10
  constraint coincident L5.end L11.end
  constraint coincident L4.start L12.start
  constraint coincident L8 L12.end
  constraint perpendicular L8 L12
  constraint coincident L2.end L3.start
  constraint coincident L8 L13.end
  constraint perpendicular L8 L13
  constraint coincident L8 P0
  constraint coincident P0 L14.start
  constraint perpendicular L8 L14
  constraint perpendicular L14 L15
  constraint midpoint L5 L16.start
  constraint coincident L8 L16.end
  constraint perpendicular L8 L16
  constraint coincident L8 L17.end
  constraint perpendicular L8 L17
  constraint tangent L15 A0
  constraint tangent L17 A0
  constraint tangent L14 A1
  constraint tangent L15 A1
  constraint equal A0 A1
  constraint coincident L8.end L9.start
  measures "d675" distance of L12.end P0
  measures "d676" distance of L5 L15
  measures "d677" distance of L13.end L17.end
  measures "d678" radius of A0
extrude "Extrude1''''''''" add sketch "Struttura" along normal blind 5 from surface at 10 separate body contours L8 L14 L15 L17 A0 A1 A2 L19 L20 | L14 A2 L19 L20 makes body 9 in component "Arpione_Struttura"
component "Arpione_Curva1" placed x (1, 0, 0) y (0, 1, 0) z (0, 0, 1) at (0, 0, 0)
component "Manopola" placed x (1, 0, 0) y (0, 1, 0) z (0, 0, 1) at (0, 0, 0)
component "Fulcro" placed x (1, 0, 0) y (0, 1, 0) z (0, 0, 1) at (0, 0, 0)
component "Cuscinetto_Basso" placed x (1, 0, 0) y (0, 1, 0) z (0, 0, 1) at (0, 0, 0)
component "Cuscinetto_Alto" placed x (1, 0, 0) y (0, 1, 0) z (0, 0, 1) at (0, 0, 0)
component "Catena" placed x (1, 0, 0) y (0, 1, 0) z (0, 0, 1) at (0, 0, 0)
component "Arpione_Curva2" placed x (1, 0, 0) y (0, 1, 0) z (0, 0, 1) at (0, 0, 0)
component "Arpione_Curva3" placed x (1, 0, 0) y (0, 1, 0) z (0, 0, 1) at (0, 0, 0)
component "Arpione_Struttura" placed x (1, 0, 0) y (0, 1, 0) z (0, 0, 1) at (0, 0, 0)
equation "d399 = 105 deg + 25 deg"
equation "d400 = d399 + 25 deg"
